Autodesk Fusion 360 part; units mm, degrees
note: some values were not read from the file. Set by a fixed rule: which sketch regions a step uses.
(part 2 of 3)
sketch "Sketch3" plane through (0, 0, 5) normal (0, 0, 1) x (-1, 0, 0)
  line L0 (-183.6113, -17.3326) -> (-182.6113, -19.0647)
  line L1 (-182.6113, -19.0647) -> (-183.6113, -20.7967)
  line L2 (-183.6113, -20.7967) -> (-179.9574, -28.2505)
  arc A0 (-179.9574, -28.2505) -> (-178.1615, -29.3702) centre (-178.1615, -27.3702) ccw
  line L3 (-178.1615, -29.3702) -> (-149.6323, -29.3702)
  line L4 (-149.6323, -29.3702) -> (-149.6323, -24.3702)
  line L5 (-149.6323, -24.3702) -> (-169.6572, -23.9078)
  arc A1 (-170.1456, -23.408) -> (-169.6572, -23.9078) centre (-169.6456, -23.408) ccw
  line L6 (-170.1456, -23.408) -> (-170.1456, -20.1187)
  arc A2 (-169.9247, -19.9198) -> (-170.1456, -20.1187) centre (-169.9456, -20.1187) ccw
  line L7 (-169.9247, -19.9198) -> (-167.3247, -20.1931)
  arc A3 (-167.1456, -20.392) -> (-167.3247, -20.1931) centre (-167.3456, -20.392) ccw
  line L8 (-167.1456, -20.392) -> (-167.1456, -20.5119)
  line L9 (-167.1456, -20.5119) -> (-151.6323, -22.1424)
  line L10 (-151.6323, -22.1424) -> (-151.6323, -22.0645)
  arc A4 (-151.4114, -21.8656) -> (-151.6323, -22.0645) centre (-151.4323, -22.0645) ccw
  line L11 (-151.4114, -21.8656) -> (-148.8114, -22.1389)
  arc A5 (-148.6323, -22.3378) -> (-148.8114, -22.1389) centre (-148.8323, -22.3378) ccw
  line L12 (-148.6323, -22.3378) -> (-148.6323, -33.3702)
  arc A6 (-149.1323, -33.8702) -> (-148.6323, -33.3702) centre (-149.1323, -33.3702) ccw
  line L13 (-149.1323, -33.8702) -> (-150.6323, -33.8702)
  arc A7 (-150.6323, -33.8702) -> (-151.1323, -34.3702) centre (-150.6323, -34.3702) ccw
  line L14 (-151.1323, -34.3702) -> (-151.1323, -38.0378)
  arc A8 (-151.1323, -38.0378) -> (-150.4871, -38.5162) centre (-150.6323, -38.0378) ccw
  arc A9 (-141.7774, -38.5162) -> (-150.4871, -38.5162) centre (-146.1323, -52.8702) ccw
  arc A10 (-141.7774, -38.5162) -> (-141.1323, -38.0378) centre (-141.6323, -38.0378) ccw
  line L15 (-141.1323, -38.0378) -> (-141.1323, -34.3702)
  arc A11 (-141.1323, -34.3702) -> (-141.6323, -33.8702) centre (-141.6323, -34.3702) ccw
  line L16 (-141.6323, -33.8702) -> (-143.1323, -33.8702)
  arc A12 (-143.6323, -33.3702) -> (-143.1323, -33.8702) centre (-143.1323, -33.3702) ccw
  line L17 (-143.6323, -33.3702) -> (-143.6323, -22.3378)
  arc A13 (-143.4532, -22.1389) -> (-143.6323, -22.3378) centre (-143.4323, -22.3378) ccw
  line L18 (-143.4532, -22.1389) -> (-140.6323, -21.8424)
  line L19 (-140.6323, -21.8424) -> (-140.6323, -21.9203)
  arc A14 (-140.6323, -21.9203) -> (-140.4114, -22.1192) centre (-140.4323, -21.9203) ccw
  line L20 (-140.4114, -22.1192) -> (-125.298, -20.5307)
  arc A15 (-125.298, -20.5307) -> (-125.1189, -20.3318) centre (-125.3189, -20.3318) ccw
  line L21 (-125.1189, -20.3318) -> (-125.1189, -20.3019)
  arc A16 (-125.0294, -20.2025) -> (-125.1189, -20.3019) centre (-125.0189, -20.3019) ccw
  line L22 (-125.0294, -20.2025) -> (-122.3398, -19.9198)
  arc A17 (-122.1189, -20.1187) -> (-122.3398, -19.9198) centre (-122.3189, -20.1187) ccw
  line L23 (-122.1189, -20.1187) -> (-122.1189, -23.408)
  arc A18 (-122.6074, -23.9078) -> (-122.1189, -23.408) centre (-122.6189, -23.408) ccw
  line L24 (-122.6074, -23.9078) -> (-142.1438, -24.3589)
  line L25 (-142.1438, -24.3589) -> (-142.6323, -24.3589)
  line L26 (-142.6323, -24.3589) -> (-142.6323, -29.3702)
  line L27 (-142.6323, -29.3702) -> (-117.7597, -29.3702)
  arc A19 (-117.7597, -29.3702) -> (-113.1229, -26.2409) centre (-117.7597, -24.3702) ccw
  arc A20 (-89.3732, -10.2649) -> (-113.1229, -26.2409) centre (-89.45, -35.7917) ccw
  line L28 (-89.3732, -10.2649) -> (-11.704, -12.452)
  arc A21 (-11.704, -12.452) -> (-11.9433, 12.5645) centre (-11.002, 0.0641) ccw
  line L29 (-11.9433, 12.5645) -> (-80.6073, 9.9709)
  arc A22 (-112.7407, 25.7315) -> (-80.6073, 9.9709) centre (-80.1774, 51.4853) ccw
  arc A23 (-112.7407, 25.7315) -> (-116.6624, 27.6298) centre (-116.6624, 22.6298) ccw
  line L30 (-116.6624, 27.6298) -> (-197.169, 27.6298)
  arc A24 (-197.169, 27.6298) -> (-202.169, 22.6429) centre (-197.169, 22.6298) ccw
  line L31 (-202.169, 22.6429) -> (-202.2039, 9.25)
  line L32 (-202.2039, 9.25) -> (-186.5961, 9.1821)
  arc A25 (-186.5961, 9.1821) -> (-186.1089, 9.5607) centre (-186.5939, 9.6821) ccw
  line L33 (-186.1089, 9.5607) -> (-182.6828, 23.2512)
  arc A26 (-182.1978, 23.6298) -> (-182.6828, 23.2512) centre (-182.1978, 23.1298) ccw
  line L34 (-182.1978, 23.6298) -> (-178.088, 23.6298)
  arc A27 (-177.588, 23.1298) -> (-178.088, 23.6298) centre (-178.088, 23.1298) ccw
  line L35 (-177.588, 23.1298) -> (-177.588, 7.1298)
  arc A28 (-178.088, 6.6298) -> (-177.588, 7.1298) centre (-178.088, 7.1298) ccw
  line L36 (-178.088, 6.6298) -> (-185.5859, 6.6298)
  arc A29 (-186.0859, 7.132) -> (-185.5859, 6.6298) centre (-185.5859, 7.1298) ccw
  line L37 (-186.0859, 7.132) -> (-186.0802, 8.4298)
  arc A30 (-186.0802, 8.4298) -> (-186.578, 8.932) centre (-186.5802, 8.432) ccw
  line L38 (-186.578, 8.932) -> (-202.156, 8.9998)
  line L39 (-202.156, 8.9998) -> (-202.156, -24.3702)
  arc A31 (-202.156, -24.3702) -> (-197.156, -29.3702) centre (-197.156, -24.3702) ccw
  line L40 (-197.156, -29.3702) -> (-190.889, -29.3702)
  arc A32 (-190.889, -29.3702) -> (-189.0932, -28.2505) centre (-190.889, -27.3702) ccw
  line L41 (-189.0932, -28.2505) -> (-185.4393, -20.7967)
  line L42 (-185.4393, -20.7967) -> (-186.4393, -19.0647)
  line L43 (-186.4393, -19.0647) -> (-185.4393, -17.3326)
  line L44 (-185.4393, -17.3326) -> (-186.4393, -15.6006)
  line L45 (-186.4393, -15.6006) -> (-185.4393, -13.8685)
  line L46 (-185.4393, -13.8685) -> (-186.4393, -12.1365)
  line L47 (-186.4393, -12.1365) -> (-185.4393, -10.4044)
  line L48 (-185.4393, -10.4044) -> (-186.4393, -8.6724)
  line L49 (-186.4393, -8.6724) -> (-185.4393, -6.9403)
  line L50 (-185.4393, -6.9403) -> (-186.4393, -5.2083)
  line L51 (-186.4393, -5.2083) -> (-185.4393, -3.4762)
  line L52 (-185.4393, -3.4762) -> (-186.4393, -1.7442)
  line L53 (-186.4393, -1.7442) -> (-185.4592, -0.0467)
  line L54 (-185.4592, -0.0467) -> (-185.4592, 2.1298)
  arc A33 (-184.9592, 2.6298) -> (-185.4592, 2.1298) centre (-184.9592, 2.1298) ccw
  line L55 (-184.9592, 2.6298) -> (-165.8788, 2.6298)
  arc A34 (-165.8788, 2.6298) -> (-165.3864, 3.043) centre (-165.8788, 3.1298) ccw
  line L56 (-165.3864, 3.043) -> (-162.9139, 17.0652)
  arc A35 (-162.4215, 17.4784) -> (-162.9139, 17.0652) centre (-162.4215, 16.9784) ccw
  line L57 (-162.4215, 17.4784) -> (-161.7176, 17.4784)
  arc A36 (-161.2489, 17.1526) -> (-161.7176, 17.4784) centre (-161.7176, 16.9784) ccw
  spline S0 degree 5 poles (-161.2489, 17.1526) (-161.0282, 16.559) (-160.5594, 15.3025) (-159.8388, 13.3845) (-158.8598, 10.8079) (-157.6127, 7.5765) (-156.3196, 4.2834) (-155.0058, 0.9987) (-153.6703, -2.2771) (-152.3141, -5.5444) (-150.9388, -8.8038) (-149.8244, -11.4057) (-148.9812, -13.354) (-148.4158, -14.6516) (-148.1323, -15.3) knots -0.989467 -0.989467 -0.989467 -0.989467 -0.989467 -0.989467 -0.9 -0.8 -0.7 -0.6 -0.5 -0.4 -0.3 -0.2 -0.1 0 0 0 0 0 0
  line L58 (-148.1323, -15.3) -> (-148.3823, -15.3)
  arc A37 (-148.3823, -15.3) -> (-148.6323, -15.55) centre (-148.3823, -15.55) ccw
  line L59 (-148.6323, -15.55) -> (-148.6323, -17.4356)
  arc A38 (-148.8532, -17.6345) -> (-148.6323, -17.4356) centre (-148.8323, -17.4356) ccw
  line L60 (-148.8532, -17.6345) -> (-151.4532, -17.3612)
  arc A39 (-151.6323, -17.1623) -> (-151.4532, -17.3612) centre (-151.4323, -17.1623) ccw
  line L61 (-151.6323, -17.1623) -> (-151.6323, -17.0424)
  line L62 (-151.6323, -17.0424) -> (-167.1456, -15.4119)
  line L63 (-167.1456, -15.4119) -> (-167.1456, -15.4898)
  arc A40 (-167.3665, -15.6887) -> (-167.1456, -15.4898) centre (-167.3456, -15.4898) ccw
  line L64 (-167.3665, -15.6887) -> (-169.9665, -15.4154)
  arc A41 (-170.1456, -15.2165) -> (-169.9665, -15.4154) centre (-169.9456, -15.2165) ccw
  line L65 (-170.1456, -15.2165) -> (-170.1456, -13.9739)
  arc A42 (-170.1456, -13.9739) -> (-170.6456, -13.1079) centre (-171.1456, -13.9739) ccw
  line L66 (-170.6456, -13.1079) -> (-173.5, -11.4599)
  arc A43 (-176, -7.1298) -> (-173.5, -11.4599) centre (-171, -7.1298) ccw
  line L67 (-176, -7.1298) -> (-176, 1.6298)
  line L68 (-176, 1.6298) -> (-183.6113, 1.6298)
  line L69 (-183.6113, 1.6298) -> (-183.6113, -0.0121)
  line L70 (-183.6113, -0.0121) -> (-182.6113, -1.7442)
  line L71 (-182.6113, -1.7442) -> (-183.6113, -3.4762)
  line L72 (-183.6113, -3.4762) -> (-182.6113, -5.2083)
  line L73 (-182.6113, -5.2083) -> (-183.6113, -6.9403)
  line L74 (-183.6113, -6.9403) -> (-182.6113, -8.6724)
  line L75 (-182.6113, -8.6724) -> (-183.6113, -10.4044)
  line L76 (-183.6113, -10.4044) -> (-182.6113, -12.1365)
  line L77 (-182.6113, -12.1365) -> (-183.6113, -13.8685)
  line L78 (-183.6113, -13.8685) -> (-182.6113, -15.6006)
  line L79 (-182.6113, -15.6006) -> (-183.6113, -17.3326)
  arc A44 (-143.6323, -21.4356) -> (-143.4114, -21.6345) centre (-143.4323, -21.4356) ccw
  line L80 (-143.6323, -21.4356) -> (-143.6323, -20.3378)
  arc A45 (-143.4532, -20.1389) -> (-143.6323, -20.3378) centre (-143.4323, -20.3378) ccw
  line L81 (-143.4532, -20.1389) -> (-140.6323, -19.8424)
  line L82 (-140.6323, -19.8424) -> (-140.6323, -19.9203)
  arc A46 (-140.6323, -19.9203) -> (-140.4114, -20.1192) centre (-140.4323, -19.9203) ccw
  line L83 (-140.4114, -20.1192) -> (-125.298, -18.5307)
  arc A47 (-125.298, -18.5307) -> (-125.1189, -18.3318) centre (-125.3189, -18.3318) ccw
  line L84 (-125.1189, -18.3318) -> (-125.1189, -18.2119)
  line L85 (-125.1189, -18.2119) -> (-122.3398, -17.9198)
  arc A48 (-122.1189, -18.1187) -> (-122.3398, -17.9198) centre (-122.3189, -18.1187) ccw
  line L86 (-122.1189, -18.1187) -> (-122.1189, -19.2165)
  arc A49 (-122.298, -19.4154) -> (-122.1189, -19.2165) centre (-122.3189, -19.2165) ccw
  line L87 (-122.298, -19.4154) -> (-125.1189, -19.7119)
  line L88 (-125.1189, -19.7119) -> (-125.1189, -19.634)
  arc A50 (-125.1189, -19.634) -> (-125.3398, -19.4351) centre (-125.3189, -19.634) ccw
  line L89 (-125.3398, -19.4351) -> (-140.4532, -21.0236)
  arc A51 (-140.4532, -21.0236) -> (-140.6323, -21.2225) centre (-140.4323, -21.2225) ccw
  line L90 (-140.6323, -21.2225) -> (-140.6323, -21.2524)
  arc A52 (-140.7218, -21.3518) -> (-140.6323, -21.2524) centre (-140.7323, -21.2524) ccw
  line L91 (-140.7218, -21.3518) -> (-143.4114, -21.6345)
  arc A53 (-143.6323, -19.4356) -> (-143.4114, -19.6345) centre (-143.4323, -19.4356) ccw
  line L92 (-143.6323, -19.4356) -> (-143.6323, -18.3378)
  arc A54 (-143.4532, -18.1389) -> (-143.6323, -18.3378) centre (-143.4323, -18.3378) ccw
  line L93 (-143.4532, -18.1389) -> (-140.6323, -17.8424)
  line L94 (-140.6323, -17.8424) -> (-140.6323, -17.9203)
  arc A55 (-140.6323, -17.9203) -> (-140.4114, -18.1192) centre (-140.4323, -17.9203) ccw
  line L95 (-140.4114, -18.1192) -> (-125.298, -16.5307)
  arc A56 (-125.298, -16.5307) -> (-125.1189, -16.3318) centre (-125.3189, -16.3318) ccw
  line L96 (-125.1189, -16.3318) -> (-125.1189, -16.2119)
  line L97 (-125.1189, -16.2119) -> (-122.3398, -15.9198)
  arc A57 (-122.1189, -16.1187) -> (-122.3398, -15.9198) centre (-122.3189, -16.1187) ccw
  line L98 (-122.1189, -16.1187) -> (-122.1189, -17.2165)
  arc A58 (-122.298, -17.4154) -> (-122.1189, -17.2165) centre (-122.3189, -17.2165) ccw
  line L99 (-122.298, -17.4154) -> (-125.1189, -17.7119)
  line L100 (-125.1189, -17.7119) -> (-125.1189, -17.634)
  arc A59 (-125.1189, -17.634) -> (-125.3398, -17.4351) centre (-125.3189, -17.634) ccw
  line L101 (-125.3398, -17.4351) -> (-140.4532, -19.0236)
  arc A60 (-140.4532, -19.0236) -> (-140.6323, -19.2225) centre (-140.4323, -19.2225) ccw
  line L102 (-140.6323, -19.2225) -> (-140.6323, -19.2524)
  arc A61 (-140.7218, -19.3518) -> (-140.6323, -19.2524) centre (-140.7323, -19.2524) ccw
  line L103 (-140.7218, -19.3518) -> (-143.4114, -19.6345)
  arc A62 (-123.4224, 7.043) -> (-122.93, 6.6298) centre (-122.93, 7.1298) ccw
  line L104 (-123.4224, 7.043) -> (-126.0097, 21.7167)
  arc A63 (-126.0097, 21.7167) -> (-126.5021, 22.1298) centre (-126.5021, 21.6298) ccw
  line L105 (-126.5021, 22.1298) -> (-165.663, 22.1298)
  arc A64 (-165.663, 22.1298) -> (-166.1554, 21.7167) centre (-165.663, 21.6298) ccw
  line L106 (-166.1554, 21.7167) -> (-168.7428, 7.043)
  arc A65 (-169.2352, 6.6298) -> (-168.7428, 7.043) centre (-169.2352, 7.1298) ccw
  line L107 (-169.2352, 6.6298) -> (-176.588, 6.6298)
  arc A66 (-177.088, 7.1298) -> (-176.588, 6.6298) centre (-176.588, 7.1298) ccw
  line L108 (-177.088, 7.1298) -> (-177.088, 23.1298)
  arc A67 (-176.588, 23.6298) -> (-177.088, 23.1298) centre (-176.588, 23.1298) ccw
  line L109 (-176.588, 23.6298) -> (-121.7059, 23.6298)
  arc A68 (-121.2059, 23.1298) -> (-121.7059, 23.6298) centre (-121.7059, 23.1298) ccw
  line L110 (-121.2059, 23.1298) -> (-121.2059, 7.1298)
  arc A69 (-121.7059, 6.6298) -> (-121.2059, 7.1298) centre (-121.7059, 7.1298) ccw
  line L111 (-121.7059, 6.6298) -> (-122.93, 6.6298)
  line L112 (-167.1456, -16.5119) -> (-151.6323, -18.1424)
  line L113 (-151.6323, -18.1424) -> (-151.6323, -18.0645)
  arc A70 (-151.4114, -17.8656) -> (-151.6323, -18.0645) centre (-151.4323, -18.0645) ccw
  line L114 (-151.4114, -17.8656) -> (-148.8114, -18.1389)
  arc A71 (-148.6323, -18.3378) -> (-148.8114, -18.1389) centre (-148.8323, -18.3378) ccw
  line L115 (-148.6323, -18.3378) -> (-148.6323, -19.4356)
  arc A72 (-148.8532, -19.6345) -> (-148.6323, -19.4356) centre (-148.8323, -19.4356) ccw
  line L116 (-148.8532, -19.6345) -> (-151.4532, -19.3612)
  arc A73 (-151.6323, -19.1623) -> (-151.4532, -19.3612) centre (-151.4323, -19.1623) ccw
  line L117 (-151.6323, -19.1623) -> (-151.6323, -19.0424)
  line L118 (-151.6323, -19.0424) -> (-167.1456, -17.4119)
  line L119 (-167.1456, -17.4119) -> (-167.1456, -17.4898)
  arc A74 (-167.3665, -17.6887) -> (-167.1456, -17.4898) centre (-167.3456, -17.4898) ccw
  line L120 (-167.3665, -17.6887) -> (-169.9665, -17.4154)
  arc A75 (-170.1456, -17.2165) -> (-169.9665, -17.4154) centre (-169.9456, -17.2165) ccw
  line L121 (-170.1456, -17.2165) -> (-170.1456, -16.1187)
  arc A76 (-169.9247, -15.9198) -> (-170.1456, -16.1187) centre (-169.9456, -16.1187) ccw
  line L122 (-169.9247, -15.9198) -> (-167.3247, -16.1931)
  arc A77 (-167.1456, -16.392) -> (-167.3247, -16.1931) centre (-167.3456, -16.392) ccw
  line L123 (-167.1456, -16.392) -> (-167.1456, -16.5119)
  spline S1 degree 5 poles (-131.6523, 17.4499) (-131.871, 16.8829) (-132.3693, 15.5934) (-133.1481, 13.5859) (-134.2095, 10.8681) (-135.5564, 7.4521) (-136.9701, 3.9054) (-138.3903, 0.385) (-139.8173, -3.108) (-141.2507, -6.5745) (-142.5604, -9.7063) (-143.5856, -12.1354) (-144.3238, -13.8732) (-144.7729, -14.9268) (-144.9323, -15.3) knots -0.978339 -0.978339 -0.978339 -0.978339 -0.978339 -0.978339 -0.9 -0.8 -0.7 -0.6 -0.5 -0.4 -0.3 -0.2 -0.1 -0.045074 -0.045074 -0.045074 -0.045074 -0.045074 -0.045074
  line L124 (-144.9323, -15.3) -> (-147.3323, -15.3)
  spline S2 degree 3 poles (-147.3323, -15.3) (-147.3606, -15.2315) (-147.3889, -15.163) (-147.4174, -15.0945) (-147.7999, -14.1733) (-148.2003, -13.2596) (-148.603, -12.3469) (-149.0343, -11.3694) (-149.4682, -10.3932) (-149.9035, -9.4176) (-150.1094, -8.9559) (-150.3157, -8.4943) (-150.5222, -8.0328) knots 80.396364 80.396364 80.396364 80.396364 80.841267 80.841267 80.841267 86.826165 86.826165 86.826165 93.23622 93.23622 93.23622 96.269727 96.269727 96.269727 96.269727
  spline S3 degree 5 poles (-150.5222, -8.0328) (-150.5836, -7.8891) (-150.9212, -7.0983) (-151.5369, -5.6459) (-152.4351, -3.5002) (-153.6231, -0.6091) (-155.0461, 2.9325) (-156.4844, 6.5848) (-157.7568, 9.8732) (-158.7459, 12.4635) (-159.4459, 14.3123) (-159.8529, 15.3927) (-159.9652, 15.6911) knots -0.722257 -0.722257 -0.722257 -0.722257 -0.722257 -0.722257 -0.7 -0.6 -0.5 -0.4 -0.3 -0.2 -0.1 -0.061951 -0.061951 -0.061951 -0.061951 -0.061951 -0.061951
  line L125 (-159.9652, 15.6911) -> (-160.6285, 17.4538)
  arc A78 (-160.1605, 18.1298) -> (-160.6285, 17.4538) centre (-160.1605, 17.6298) ccw
  line L126 (-160.1605, 18.1298) -> (-132.1188, 18.1298)
  arc A79 (-131.6523, 17.4499) -> (-132.1188, 18.1298) centre (-132.1188, 17.6298) ccw
  arc A80 (-143.6323, -17.4356) -> (-143.4114, -17.6345) centre (-143.4323, -17.4356) ccw
  line L127 (-143.6323, -17.4356) -> (-143.6323, -15.55)
  arc A81 (-143.6323, -15.55) -> (-143.8823, -15.3) centre (-143.8823, -15.55) ccw
  line L128 (-143.8823, -15.3) -> (-144.1323, -15.3)
  spline S4 degree 5 poles (-144.1323, -15.3) (-144.0034, -15.0117) (-143.5692, -14.0387) (-142.8329, -12.3782) (-141.8006, -10.0246) (-140.482, -6.9691) (-139.0131, -3.4934) (-137.5684, 0.0041) (-136.1486, 3.5243) (-134.7528, 7.0662) (-133.3923, 10.5941) (-132.3224, 13.424) (-131.5314, 15.5453) (-131.012, 16.9513) (-130.7595, 17.6378) knots -0.94214 -0.94214 -0.94214 -0.94214 -0.94214 -0.94214 -0.9 -0.8 -0.7 -0.6 -0.5 -0.4 -0.3 -0.2 -0.1 -0.004792 -0.004792 -0.004792 -0.004792 -0.004792 -0.004792
  line L129 (-130.7595, 17.6378) -> (-129.7718, 17.6378)
  arc A82 (-129.2794, 17.2246) -> (-129.7718, 17.6378) centre (-129.7718, 17.1378) ccw
  line L130 (-129.2794, 17.2246) -> (-126.7788, 3.043)
  arc A83 (-126.7788, 3.043) -> (-126.2864, 2.6298) centre (-126.2864, 3.1298) ccw
  line L131 (-126.2864, 2.6298) -> (-120.2059, 2.6298)
  arc A84 (-120.2059, 2.6298) -> (-119.7059, 3.1298) centre (-120.2059, 3.1298) ccw
  line L132 (-119.7059, 3.1298) -> (-119.7059, 6.1298)
  arc A85 (-119.7059, 6.1298) -> (-120.2059, 6.6298) centre (-120.2059, 6.1298) ccw
  arc A86 (-120.7059, 7.1298) -> (-120.2059, 6.6298) centre (-120.2059, 7.1298) ccw
  line L133 (-120.7059, 7.1298) -> (-120.7059, 23.1298)
  arc A87 (-120.2059, 23.6298) -> (-120.7059, 23.1298) centre (-120.2059, 23.1298) ccw
  line L134 (-120.2059, 23.6298) -> (-118.121, 23.6298)
  arc A88 (-117.6301, 23.2247) -> (-118.121, 23.6298) centre (-118.121, 23.1298) ccw
  line L135 (-117.6301, 23.2247) -> (-115.2816, 11.0735)
  line L136 (-115.1907, 10.1247) -> (-115.1907, -6.5098)
  arc A89 (-117.6907, -10.8399) -> (-115.1907, -6.5098) centre (-120.1907, -6.5098) ccw
  line L137 (-117.6907, -10.8399) -> (-121.6189, -13.1079)
  arc A90 (-121.6189, -13.1079) -> (-122.1189, -13.9739) centre (-121.1189, -13.9739) ccw
  line L138 (-122.1189, -13.9739) -> (-122.1189, -15.2165)
  arc A91 (-122.298, -15.4154) -> (-122.1189, -15.2165) centre (-122.3189, -15.2165) ccw
  line L139 (-122.298, -15.4154) -> (-125.1189, -15.7119)
  line L140 (-125.1189, -15.7119) -> (-125.1189, -15.634)
  arc A92 (-125.1189, -15.634) -> (-125.3398, -15.4351) centre (-125.3189, -15.634) ccw
  line L141 (-125.3398, -15.4351) -> (-140.4532, -17.0236)
  arc A93 (-140.4532, -17.0236) -> (-140.6323, -17.2225) centre (-140.4323, -17.2225) ccw
  line L142 (-140.6323, -17.2225) -> (-140.6323, -17.1623)
  arc A94 (-140.8114, -17.3612) -> (-140.6323, -17.1623) centre (-140.8323, -17.1623) ccw
  line L143 (-140.8114, -17.3612) -> (-143.4114, -17.6345)
  line L144 (-167.1456, -18.5119) -> (-151.6323, -20.1424)
  line L145 (-151.6323, -20.1424) -> (-151.6323, -20.0645)
  arc A95 (-151.4114, -19.8656) -> (-151.6323, -20.0645) centre (-151.4323, -20.0645) ccw
  line L146 (-151.4114, -19.8656) -> (-148.8114, -20.1389)
  arc A96 (-148.6323, -20.3378) -> (-148.8114, -20.1389) centre (-148.8323, -20.3378) ccw
  line L147 (-148.6323, -20.3378) -> (-148.6323, -21.4356)
  arc A97 (-148.8532, -21.6345) -> (-148.6323, -21.4356) centre (-148.8323, -21.4356) ccw
  line L148 (-148.8532, -21.6345) -> (-151.4532, -21.3612)
  arc A98 (-151.6323, -21.1623) -> (-151.4532, -21.3612) centre (-151.4323, -21.1623) ccw
  line L149 (-151.6323, -21.1623) -> (-151.6323, -21.0424)
  line L150 (-151.6323, -21.0424) -> (-167.1456, -19.4119)
  line L151 (-167.1456, -19.4119) -> (-167.1456, -19.4898)
  arc A99 (-167.3665, -19.6887) -> (-167.1456, -19.4898) centre (-167.3456, -19.4898) ccw
  line L152 (-167.3665, -19.6887) -> (-169.9665, -19.4154)
  arc A100 (-170.1456, -19.2165) -> (-169.9665, -19.4154) centre (-169.9456, -19.2165) ccw
  line L153 (-170.1456, -19.2165) -> (-170.1456, -18.1187)
  arc A101 (-169.9247, -17.9198) -> (-170.1456, -18.1187) centre (-169.9456, -18.1187) ccw
  line L154 (-169.9247, -17.9198) -> (-167.3247, -18.1931)
  arc A102 (-167.1456, -18.392) -> (-167.3247, -18.1931) centre (-167.3456, -18.392) ccw
  line L155 (-167.1456, -18.392) -> (-167.1456, -18.5119)
  circle A103 centre (-11.002, 0.0641) radius 7.5
  line L156 (-126.9683, -24.0085) -> (-126.9683, -29.3702)
  line L157 (-164.0862, -24.0085) -> (-164.0862, -29.3702)
  line L158 (-182.6113, -5.2083) -> (-178.6113, -5.2083)
  line L159 (-178.6113, -5.2083) -> (-178.6113, 1.6298)
  arc A104 (-115.1907, 10.1247) -> (-115.2816, 11.0735) centre (-120.1907, 10.1247) ccw
  dimension "d155" = 5
  constraint coincident L24 L156.start
  constraint coincident L27 L156.end
  constraint perpendicular L27 L156
  constraint coincident L3 L157.end
  constraint perpendicular L3 L157
  constraint coincident L72.end L73.start
  constraint perpendicular L67 L158
  constraint coincident L68 L159.end
  constraint perpendicular L68 L159
  measures "d155" distance of L69 L159
extrude "Extrude2" add sketch "Sketch3" along normal blind 2 contours L3 L4 L5 L157 | L68 L69 L70 L71 L72 L158 L159 | L24 L25 L26 L27 L156
sketch "Sketch4" plane through (0, -1.6298, 0) normal (0, -1, 0) x (1, 0, 0)
  line L0 (176, 0) -> (183.6113, 0)
  line L1 (183.6113, 0) -> (183.6113, 7)
  line L2 (183.6113, 7) -> (178.6113, 7)
  line L3 (178.6113, 7) -> (178.6113, 5)
  line L4 (178.6113, 5) -> (176, 5)
  line L5 (176, 5) -> (176, 0)
  line L6 (178.6113, 7) -> (183.6113, 7)
  line L7 (183.6113, 7) -> (183.6113, 5.3)
  line L8 (183.6113, 5.3) -> (178.6113, 5.3)
  line L9 (178.6113, 5.3) -> (178.6113, 7)
  dimension "d156" = 1.7
  constraint horizontal L6
  constraint vertical L7
  constraint horizontal L8
  constraint vertical L9
  constraint coincident L2.end L3.start
  measures "d156" distance of L2.end L8.end
sketch "Sketch5" plane through (149.6323, 0, 0) normal (-1, 0, 0) x (0, -1, 0)
  line L0 (-29.3702, 0) -> (-24.3702, 0)
  line L1 (-24.3702, 0) -> (-24.3702, 7)
  line L2 (-24.3702, 7) -> (-29.3702, 7)
  line L3 (-29.3702, 7) -> (-29.3702, 0)
  line L4 (-29.3702, 7) -> (-24.3702, 7)
  line L5 (-24.3702, 7) -> (-24.3702, 5.3)
  line L6 (-24.3702, 5.3) -> (-29.3702, 5.3)
  line L7 (-29.3702, 5.3) -> (-29.3702, 7)
  dimension "d157" = 1.7
  constraint horizontal L4
  constraint vertical L5
  constraint horizontal L6
  constraint vertical L7
  constraint coincident L2.end L3.start
  measures "d157" distance of L2.end L6.end
extrude "Extrude3" add sketch "Sketch5" along normal blind 7 contours L1 L2 L3 L4 L5 L6 L7
extrude "Extrude4" add sketch "Sketch4" along normal blind 26 contours L1 L2 L3 L6 L7 L8 L9
sketch "Sketch6" plane through (0, 0, 5) normal (0, 0, 1) x (-1, 0, 0)
  line L0 (-178.6113, 1.6298) -> (-178.6113, -5.2083)
  line L1 (-178.6113, -5.2083) -> (-182.6113, -5.2083)
  line L2 (-182.6113, -5.2083) -> (-183.6113, -6.9403)
  line L3 (-183.6113, -6.9403) -> (-182.6113, -8.6724)
  line L4 (-182.6113, -8.6724) -> (-183.6113, -10.4044)
  line L5 (-183.6113, -10.4044) -> (-182.6113, -12.1365)
  line L6 (-182.6113, -12.1365) -> (-183.6113, -13.8685)
  line L7 (-183.6113, -13.8685) -> (-182.6113, -15.6006)
  line L8 (-182.6113, -15.6006) -> (-183.6113, -17.3326)
  line L9 (-183.6113, -17.3326) -> (-182.6113, -19.0647)
  line L10 (-182.6113, -19.0647) -> (-183.6113, -20.7967)
  line L11 (-183.6113, -20.7967) -> (-179.9574, -28.2505)
  arc A0 (-179.9574, -28.2505) -> (-178.1615, -29.3702) centre (-178.1615, -27.3702) ccw
  line L12 (-178.1615, -29.3702) -> (-164.0862, -29.3702)
  line L13 (-164.0862, -29.3702) -> (-164.0862, -24.0365)
  line L14 (-164.0862, -24.0365) -> (-169.6572, -23.9078)
  arc A1 (-170.1456, -23.408) -> (-169.6572, -23.9078) centre (-169.6456, -23.408) ccw
  line L15 (-170.1456, -23.408) -> (-170.1456, -20.1187)
  arc A2 (-169.9247, -19.9198) -> (-170.1456, -20.1187) centre (-169.9456, -20.1187) ccw
  line L16 (-169.9247, -19.9198) -> (-167.3247, -20.1931)
  arc A3 (-167.1456, -20.392) -> (-167.3247, -20.1931) centre (-167.3456, -20.392) ccw
  line L17 (-167.1456, -20.392) -> (-167.1456, -20.5119)
  line L18 (-167.1456, -20.5119) -> (-151.6323, -22.1424)
  line L19 (-151.6323, -22.1424) -> (-151.6323, -22.0645)
  arc A4 (-151.4114, -21.8656) -> (-151.6323, -22.0645) centre (-151.4323, -22.0645) ccw
  line L20 (-151.4114, -21.8656) -> (-148.8114, -22.1389)
  arc A5 (-148.6323, -22.3378) -> (-148.8114, -22.1389) centre (-148.8323, -22.3378) ccw
  line L21 (-148.6323, -22.3378) -> (-148.6323, -33.3702)
  arc A6 (-149.1323, -33.8702) -> (-148.6323, -33.3702) centre (-149.1323, -33.3702) ccw
  line L22 (-149.1323, -33.8702) -> (-150.6323, -33.8702)
  arc A7 (-150.6323, -33.8702) -> (-151.1323, -34.3702) centre (-150.6323, -34.3702) ccw
  line L23 (-151.1323, -34.3702) -> (-151.1323, -38.0378)
  arc A8 (-151.1323, -38.0378) -> (-150.4871, -38.5162) centre (-150.6323, -38.0378) ccw
  arc A9 (-141.7774, -38.5162) -> (-150.4871, -38.5162) centre (-146.1323, -52.8702) ccw
  arc A10 (-141.7774, -38.5162) -> (-141.1323, -38.0378) centre (-141.6323, -38.0378) ccw
  line L24 (-141.1323, -38.0378) -> (-141.1323, -34.3702)
  arc A11 (-141.1323, -34.3702) -> (-141.6323, -33.8702) centre (-141.6323, -34.3702) ccw
  line L25 (-141.6323, -33.8702) -> (-143.1323, -33.8702)
  arc A12 (-143.6323, -33.3702) -> (-143.1323, -33.8702) centre (-143.1323, -33.3702) ccw
  line L26 (-143.6323, -33.3702) -> (-143.6323, -22.3378)
  arc A13 (-143.4532, -22.1389) -> (-143.6323, -22.3378) centre (-143.4323, -22.3378) ccw
  line L27 (-143.4532, -22.1389) -> (-140.6323, -21.8424)
  line L28 (-140.6323, -21.8424) -> (-140.6323, -21.9203)
  arc A14 (-140.6323, -21.9203) -> (-140.4114, -22.1192) centre (-140.4323, -21.9203) ccw
  line L29 (-140.4114, -22.1192) -> (-125.298, -20.5307)
  arc A15 (-125.298, -20.5307) -> (-125.1189, -20.3318) centre (-125.3189, -20.3318) ccw
  line L30 (-125.1189, -20.3318) -> (-125.1189, -20.3019)
  arc A16 (-125.0294, -20.2025) -> (-125.1189, -20.3019) centre (-125.0189, -20.3019) ccw
  line L31 (-125.0294, -20.2025) -> (-122.3398, -19.9198)
  arc A17 (-122.1189, -20.1187) -> (-122.3398, -19.9198) centre (-122.3189, -20.1187) ccw
  line L32 (-122.1189, -20.1187) -> (-122.1189, -23.408)
  arc A18 (-122.6074, -23.9078) -> (-122.1189, -23.408) centre (-122.6189, -23.408) ccw
  line L33 (-122.6074, -23.9078) -> (-126.9683, -24.0085)
  line L34 (-126.9683, -24.0085) -> (-126.9683, -29.3702)
  line L35 (-126.9683, -29.3702) -> (-117.7597, -29.3702)
  arc A19 (-117.7597, -29.3702) -> (-113.1229, -26.2409) centre (-117.7597, -24.3702) ccw
  arc A20 (-89.3732, -10.2649) -> (-113.1229, -26.2409) centre (-89.45, -35.7917) ccw
  line L36 (-89.3732, -10.2649) -> (-11.704, -12.452)
  arc A21 (-11.704, -12.452) -> (-11.9433, 12.5645) centre (-11.002, 0.0641) ccw
  line L37 (-11.9433, 12.5645) -> (-80.6073, 9.9709)
  arc A22 (-112.7407, 25.7315) -> (-80.6073, 9.9709) centre (-80.1774, 51.4853) ccw
  arc A23 (-112.7407, 25.7315) -> (-116.6624, 27.6298) centre (-116.6624, 22.6298) ccw
  line L38 (-116.6624, 27.6298) -> (-197.169, 27.6298)
  arc A24 (-197.169, 27.6298) -> (-202.169, 22.6429) centre (-197.169, 22.6298) ccw
  line L39 (-202.169, 22.6429) -> (-202.2039, 9.25)
  line L40 (-202.2039, 9.25) -> (-186.5961, 9.1821)
  arc A25 (-186.5961, 9.1821) -> (-186.1089, 9.5607) centre (-186.5939, 9.6821) ccw
  line L41 (-186.1089, 9.5607) -> (-182.6828, 23.2512)
  arc A26 (-182.1978, 23.6298) -> (-182.6828, 23.2512) centre (-182.1978, 23.1298) ccw
  line L42 (-182.1978, 23.6298) -> (-178.088, 23.6298)
  arc A27 (-177.588, 23.1298) -> (-178.088, 23.6298) centre (-178.088, 23.1298) ccw
  line L43 (-177.588, 23.1298) -> (-177.588, 7.1298)
  arc A28 (-178.088, 6.6298) -> (-177.588, 7.1298) centre (-178.088, 7.1298) ccw
  line L44 (-178.088, 6.6298) -> (-185.5859, 6.6298)
  arc A29 (-186.0859, 7.132) -> (-185.5859, 6.6298) centre (-185.5859, 7.1298) ccw
  line L45 (-186.0859, 7.132) -> (-186.0802, 8.4298)
  arc A30 (-186.0802, 8.4298) -> (-186.578, 8.932) centre (-186.5802, 8.432) ccw
  line L46 (-186.578, 8.932) -> (-202.156, 8.9998)
  line L47 (-202.156, 8.9998) -> (-202.156, -24.3702)
  arc A31 (-202.156, -24.3702) -> (-197.156, -29.3702) centre (-197.156, -24.3702) ccw
  line L48 (-197.156, -29.3702) -> (-190.889, -29.3702)
  arc A32 (-190.889, -29.3702) -> (-189.0932, -28.2505) centre (-190.889, -27.3702) ccw
  line L49 (-189.0932, -28.2505) -> (-185.4393, -20.7967)
  line L50 (-185.4393, -20.7967) -> (-186.4393, -19.0647)
  line L51 (-186.4393, -19.0647) -> (-185.4393, -17.3326)
  line L52 (-185.4393, -17.3326) -> (-186.4393, -15.6006)
  line L53 (-186.4393, -15.6006) -> (-185.4393, -13.8685)
  line L54 (-185.4393, -13.8685) -> (-186.4393, -12.1365)
  line L55 (-186.4393, -12.1365) -> (-185.4393, -10.4044)
  line L56 (-185.4393, -10.4044) -> (-186.4393, -8.6724)
  line L57 (-186.4393, -8.6724) -> (-185.4393, -6.9403)
  line L58 (-185.4393, -6.9403) -> (-186.4393, -5.2083)
  line L59 (-186.4393, -5.2083) -> (-185.4393, -3.4762)
  line L60 (-185.4393, -3.4762) -> (-186.4393, -1.7442)
  line L61 (-186.4393, -1.7442) -> (-185.4592, -0.0467)
  line L62 (-185.4592, -0.0467) -> (-185.4592, 2.1298)
  arc A33 (-184.9592, 2.6298) -> (-185.4592, 2.1298) centre (-184.9592, 2.1298) ccw
  line L63 (-184.9592, 2.6298) -> (-165.8788, 2.6298)
  arc A34 (-165.8788, 2.6298) -> (-165.3864, 3.043) centre (-165.8788, 3.1298) ccw
  line L64 (-165.3864, 3.043) -> (-162.9139, 17.0652)
  arc A35 (-162.4215, 17.4784) -> (-162.9139, 17.0652) centre (-162.4215, 16.9784) ccw
  line L65 (-162.4215, 17.4784) -> (-161.7176, 17.4784)
  arc A36 (-161.2489, 17.1526) -> (-161.7176, 17.4784) centre (-161.7176, 16.9784) ccw
  spline S0 degree 5 poles (-161.2489, 17.1526) (-161.0282, 16.559) (-160.5594, 15.3025) (-159.8388, 13.3845) (-158.8598, 10.8079) (-157.6127, 7.5765) (-156.3196, 4.2834) (-155.0058, 0.9987) (-153.6703, -2.2771) (-152.3141, -5.5444) (-150.9388, -8.8038) (-149.8244, -11.4057) (-148.9812, -13.354) (-148.4158, -14.6516) (-148.1323, -15.3) knots -0.989467 -0.989467 -0.989467 -0.989467 -0.989467 -0.989467 -0.9 -0.8 -0.7 -0.6 -0.5 -0.4 -0.3 -0.2 -0.1 0 0 0 0 0 0
  line L66 (-148.1323, -15.3) -> (-148.3823, -15.3)
  arc A37 (-148.3823, -15.3) -> (-148.6323, -15.55) centre (-148.3823, -15.55) ccw
  line L67 (-148.6323, -15.55) -> (-148.6323, -17.4356)
  arc A38 (-148.8532, -17.6345) -> (-148.6323, -17.4356) centre (-148.8323, -17.4356) ccw
  line L68 (-148.8532, -17.6345) -> (-151.4532, -17.3612)
  arc A39 (-151.6323, -17.1623) -> (-151.4532, -17.3612) centre (-151.4323, -17.1623) ccw
  line L69 (-151.6323, -17.1623) -> (-151.6323, -17.0424)
  line L70 (-151.6323, -17.0424) -> (-167.1456, -15.4119)
  line L71 (-167.1456, -15.4119) -> (-167.1456, -15.4898)
  arc A40 (-167.3665, -15.6887) -> (-167.1456, -15.4898) centre (-167.3456, -15.4898) ccw
  line L72 (-167.3665, -15.6887) -> (-169.9665, -15.4154)
  arc A41 (-170.1456, -15.2165) -> (-169.9665, -15.4154) centre (-169.9456, -15.2165) ccw
  line L73 (-170.1456, -15.2165) -> (-170.1456, -13.9739)
  arc A42 (-170.1456, -13.9739) -> (-170.6456, -13.1079) centre (-171.1456, -13.9739) ccw
  line L74 (-170.6456, -13.1079) -> (-173.5, -11.4599)
  arc A43 (-176, -7.1298) -> (-173.5, -11.4599) centre (-171, -7.1298) ccw
  line L75 (-176, -7.1298) -> (-176, 1.6298)
  line L76 (-176, 1.6298) -> (-178.6113, 1.6298)
  circle A44 centre (-11.002, 0.0641) radius 7.5
  line L77 (-167.1456, -18.5119) -> (-151.6323, -20.1424)
  line L78 (-151.6323, -20.1424) -> (-151.6323, -20.0645)
  arc A45 (-151.4114, -19.8656) -> (-151.6323, -20.0645) centre (-151.4323, -20.0645) ccw
  line L79 (-151.4114, -19.8656) -> (-148.8114, -20.1389)
  arc A46 (-148.6323, -20.3378) -> (-148.8114, -20.1389) centre (-148.8323, -20.3378) ccw
  line L80 (-148.6323, -20.3378) -> (-148.6323, -21.4356)
  arc A47 (-148.8532, -21.6345) -> (-148.6323, -21.4356) centre (-148.8323, -21.4356) ccw
  line L81 (-148.8532, -21.6345) -> (-151.4532, -21.3612)
  arc A48 (-151.6323, -21.1623) -> (-151.4532, -21.3612) centre (-151.4323, -21.1623) ccw
  line L82 (-151.6323, -21.1623) -> (-151.6323, -21.0424)
  line L83 (-151.6323, -21.0424) -> (-167.1456, -19.4119)
  line L84 (-167.1456, -19.4119) -> (-167.1456, -19.4898)
  arc A49 (-167.3665, -19.6887) -> (-167.1456, -19.4898) centre (-167.3456, -19.4898) ccw
  line L85 (-167.3665, -19.6887) -> (-169.9665, -19.4154)
  arc A50 (-170.1456, -19.2165) -> (-169.9665, -19.4154) centre (-169.9456, -19.2165) ccw
  line L86 (-170.1456, -19.2165) -> (-170.1456, -18.1187)
  arc A51 (-169.9247, -17.9198) -> (-170.1456, -18.1187) centre (-169.9456, -18.1187) ccw
  line L87 (-169.9247, -17.9198) -> (-167.3247, -18.1931)
  arc A52 (-167.1456, -18.392) -> (-167.3247, -18.1931) centre (-167.3456, -18.392) ccw
  line L88 (-167.1456, -18.392) -> (-167.1456, -18.5119)
  arc A53 (-143.6323, -17.4356) -> (-143.4114, -17.6345) centre (-143.4323, -17.4356) ccw
  line L89 (-143.6323, -17.4356) -> (-143.6323, -15.55)
  arc A54 (-143.6323, -15.55) -> (-143.8823, -15.3) centre (-143.8823, -15.55) ccw
  line L90 (-143.8823, -15.3) -> (-144.1323, -15.3)
  spline S1 degree 5 poles (-144.1323, -15.3) (-144.0034, -15.0117) (-143.5692, -14.0387) (-142.8329, -12.3782) (-141.8006, -10.0246) (-140.482, -6.9691) (-139.0131, -3.4934) (-137.5684, 0.0041) (-136.1486, 3.5243) (-134.7528, 7.0662) (-133.3923, 10.5941) (-132.3224, 13.424) (-131.5314, 15.5453) (-131.012, 16.9513) (-130.7595, 17.6378) knots -0.94214 -0.94214 -0.94214 -0.94214 -0.94214 -0.94214 -0.9 -0.8 -0.7 -0.6 -0.5 -0.4 -0.3 -0.2 -0.1 -0.004792 -0.004792 -0.004792 -0.004792 -0.004792 -0.004792
  line L91 (-130.7595, 17.6378) -> (-129.7718, 17.6378)
  arc A55 (-129.2794, 17.2246) -> (-129.7718, 17.6378) centre (-129.7718, 17.1378) ccw
  line L92 (-129.2794, 17.2246) -> (-126.7788, 3.043)
  arc A56 (-126.7788, 3.043) -> (-126.2864, 2.6298) centre (-126.2864, 3.1298) ccw
  line L93 (-126.2864, 2.6298) -> (-120.2059, 2.6298)
  arc A57 (-120.2059, 2.6298) -> (-119.7059, 3.1298) centre (-120.2059, 3.1298) ccw
  line L94 (-119.7059, 3.1298) -> (-119.7059, 6.1298)
  arc A58 (-119.7059, 6.1298) -> (-120.2059, 6.6298) centre (-120.2059, 6.1298) ccw
  arc A59 (-120.7059, 7.1298) -> (-120.2059, 6.6298) centre (-120.2059, 7.1298) ccw
  line L95 (-120.7059, 7.1298) -> (-120.7059, 23.1298)
  arc A60 (-120.2059, 23.6298) -> (-120.7059, 23.1298) centre (-120.2059, 23.1298) ccw
  line L96 (-120.2059, 23.6298) -> (-118.121, 23.6298)
  arc A61 (-117.6301, 23.2247) -> (-118.121, 23.6298) centre (-118.121, 23.1298) ccw
  line L97 (-117.6301, 23.2247) -> (-115.2816, 11.0735)
  line L98 (-115.1907, 10.1247) -> (-115.1907, -6.5098)
  arc A62 (-117.6907, -10.8399) -> (-115.1907, -6.5098) centre (-120.1907, -6.5098) ccw
  line L99 (-117.6907, -10.8399) -> (-121.6189, -13.1079)
  arc A63 (-121.6189, -13.1079) -> (-122.1189, -13.9739) centre (-121.1189, -13.9739) ccw
  line L100 (-122.1189, -13.9739) -> (-122.1189, -15.2165)
  arc A64 (-122.298, -15.4154) -> (-122.1189, -15.2165) centre (-122.3189, -15.2165) ccw
  line L101 (-122.298, -15.4154) -> (-125.1189, -15.7119)
  line L102 (-125.1189, -15.7119) -> (-125.1189, -15.634)
  arc A65 (-125.1189, -15.634) -> (-125.3398, -15.4351) centre (-125.3189, -15.634) ccw
  line L103 (-125.3398, -15.4351) -> (-140.4532, -17.0236)
  arc A66 (-140.4532, -17.0236) -> (-140.6323, -17.2225) centre (-140.4323, -17.2225) ccw
  line L104 (-140.6323, -17.2225) -> (-140.6323, -17.1623)
  arc A67 (-140.8114, -17.3612) -> (-140.6323, -17.1623) centre (-140.8323, -17.1623) ccw
  line L105 (-140.8114, -17.3612) -> (-143.4114, -17.6345)
  spline S2 degree 5 poles (-131.6523, 17.4499) (-131.871, 16.8829) (-132.3693, 15.5934) (-133.1481, 13.5859) (-134.2095, 10.8681) (-135.5564, 7.4521) (-136.9701, 3.9054) (-138.3903, 0.385) (-139.8173, -3.108) (-141.2507, -6.5745) (-142.5604, -9.7063) (-143.5856, -12.1354) (-144.3238, -13.8732) (-144.7729, -14.9268) (-144.9323, -15.3) knots -0.978339 -0.978339 -0.978339 -0.978339 -0.978339 -0.978339 -0.9 -0.8 -0.7 -0.6 -0.5 -0.4 -0.3 -0.2 -0.1 -0.045074 -0.045074 -0.045074 -0.045074 -0.045074 -0.045074
  line L106 (-144.9323, -15.3) -> (-147.3323, -15.3)
  spline S3 degree 3 poles (-147.3323, -15.3) (-147.3606, -15.2315) (-147.3889, -15.163) (-147.4174, -15.0945) (-147.7999, -14.1733) (-148.2003, -13.2596) (-148.603, -12.3469) (-149.0343, -11.3694) (-149.4682, -10.3932) (-149.9035, -9.4176) (-150.1094, -8.9559) (-150.3157, -8.4943) (-150.5222, -8.0328) knots 80.396364 80.396364 80.396364 80.396364 80.841267 80.841267 80.841267 86.826165 86.826165 86.826165 93.23622 93.23622 93.23622 96.269727 96.269727 96.269727 96.269727
  spline S4 degree 5 poles (-150.5222, -8.0328) (-150.5836, -7.8891) (-150.9212, -7.0983) (-151.5369, -5.6459) (-152.4351, -3.5002) (-153.6231, -0.6091) (-155.0461, 2.9325) (-156.4844, 6.5848) (-157.7568, 9.8732) (-158.7459, 12.4635) (-159.4459, 14.3123) (-159.8529, 15.3927) (-159.9652, 15.6911) knots -0.722257 -0.722257 -0.722257 -0.722257 -0.722257 -0.722257 -0.7 -0.6 -0.5 -0.4 -0.3 -0.2 -0.1 -0.061951 -0.061951 -0.061951 -0.061951 -0.061951 -0.061951
  line L107 (-159.9652, 15.6911) -> (-160.6285, 17.4538)
  arc A68 (-160.1605, 18.1298) -> (-160.6285, 17.4538) centre (-160.1605, 17.6298) ccw
  line L108 (-160.1605, 18.1298) -> (-132.1188, 18.1298)
  arc A69 (-131.6523, 17.4499) -> (-132.1188, 18.1298) centre (-132.1188, 17.6298) ccw
  line L109 (-167.1456, -16.5119) -> (-151.6323, -18.1424)
  line L110 (-151.6323, -18.1424) -> (-151.6323, -18.0645)
  arc A70 (-151.4114, -17.8656) -> (-151.6323, -18.0645) centre (-151.4323, -18.0645) ccw
  line L111 (-151.4114, -17.8656) -> (-148.8114, -18.1389)
  arc A71 (-148.6323, -18.3378) -> (-148.8114, -18.1389) centre (-148.8323, -18.3378) ccw
  line L112 (-148.6323, -18.3378) -> (-148.6323, -19.4356)
  arc A72 (-148.8532, -19.6345) -> (-148.6323, -19.4356) centre (-148.8323, -19.4356) ccw
  line L113 (-148.8532, -19.6345) -> (-151.4532, -19.3612)
  arc A73 (-151.6323, -19.1623) -> (-151.4532, -19.3612) centre (-151.4323, -19.1623) ccw
  line L114 (-151.6323, -19.1623) -> (-151.6323, -19.0424)
  line L115 (-151.6323, -19.0424) -> (-167.1456, -17.4119)
  line L116 (-167.1456, -17.4119) -> (-167.1456, -17.4898)
  arc A74 (-167.3665, -17.6887) -> (-167.1456, -17.4898) centre (-167.3456, -17.4898) ccw
  line L117 (-167.3665, -17.6887) -> (-169.9665, -17.4154)
  arc A75 (-170.1456, -17.2165) -> (-169.9665, -17.4154) centre (-169.9456, -17.2165) ccw
  line L118 (-170.1456, -17.2165) -> (-170.1456, -16.1187)
  arc A76 (-169.9247, -15.9198) -> (-170.1456, -16.1187) centre (-169.9456, -16.1187) ccw
  line L119 (-169.9247, -15.9198) -> (-167.3247, -16.1931)
  arc A77 (-167.1456, -16.392) -> (-167.3247, -16.1931) centre (-167.3456, -16.392) ccw
  line L120 (-167.1456, -16.392) -> (-167.1456, -16.5119)
  arc A78 (-123.4224, 7.043) -> (-122.93, 6.6298) centre (-122.93, 7.1298) ccw
  line L121 (-123.4224, 7.043) -> (-126.0097, 21.7167)
  arc A79 (-126.0097, 21.7167) -> (-126.5021, 22.1298) centre (-126.5021, 21.6298) ccw
  line L122 (-126.5021, 22.1298) -> (-165.663, 22.1298)
  arc A80 (-165.663, 22.1298) -> (-166.1554, 21.7167) centre (-165.663, 21.6298) ccw
  line L123 (-166.1554, 21.7167) -> (-168.7428, 7.043)
  arc A81 (-169.2352, 6.6298) -> (-168.7428, 7.043) centre (-169.2352, 7.1298) ccw
  line L124 (-169.2352, 6.6298) -> (-176.588, 6.6298)
  arc A82 (-177.088, 7.1298) -> (-176.588, 6.6298) centre (-176.588, 7.1298) ccw
  line L125 (-177.088, 7.1298) -> (-177.088, 23.1298)
  arc A83 (-176.588, 23.6298) -> (-177.088, 23.1298) centre (-176.588, 23.1298) ccw
  line L126 (-176.588, 23.6298) -> (-121.7059, 23.6298)
  arc A84 (-121.2059, 23.1298) -> (-121.7059, 23.6298) centre (-121.7059, 23.1298) ccw
  line L127 (-121.2059, 23.1298) -> (-121.2059, 7.1298)
  arc A85 (-121.7059, 6.6298) -> (-121.2059, 7.1298) centre (-121.7059, 7.1298) ccw
  line L128 (-121.7059, 6.6298) -> (-122.93, 6.6298)
  arc A86 (-143.6323, -19.4356) -> (-143.4114, -19.6345) centre (-143.4323, -19.4356) ccw
  line L129 (-143.6323, -19.4356) -> (-143.6323, -18.3378)
  arc A87 (-143.4532, -18.1389) -> (-143.6323, -18.3378) centre (-143.4323, -18.3378) ccw
  line L130 (-143.4532, -18.1389) -> (-140.6323, -17.8424)
  line L131 (-140.6323, -17.8424) -> (-140.6323, -17.9203)
  arc A88 (-140.6323, -17.9203) -> (-140.4114, -18.1192) centre (-140.4323, -17.9203) ccw
  line L132 (-140.4114, -18.1192) -> (-125.298, -16.5307)
  arc A89 (-125.298, -16.5307) -> (-125.1189, -16.3318) centre (-125.3189, -16.3318) ccw
  line L133 (-125.1189, -16.3318) -> (-125.1189, -16.2119)
  line L134 (-125.1189, -16.2119) -> (-122.3398, -15.9198)
  arc A90 (-122.1189, -16.1187) -> (-122.3398, -15.9198) centre (-122.3189, -16.1187) ccw
  line L135 (-122.1189, -16.1187) -> (-122.1189, -17.2165)
  arc A91 (-122.298, -17.4154) -> (-122.1189, -17.2165) centre (-122.3189, -17.2165) ccw
  line L136 (-122.298, -17.4154) -> (-125.1189, -17.7119)
  line L137 (-125.1189, -17.7119) -> (-125.1189, -17.634)
  arc A92 (-125.1189, -17.634) -> (-125.3398, -17.4351) centre (-125.3189, -17.634) ccw
  line L138 (-125.3398, -17.4351) -> (-140.4532, -19.0236)
  arc A93 (-140.4532, -19.0236) -> (-140.6323, -19.2225) centre (-140.4323, -19.2225) ccw
  line L139 (-140.6323, -19.2225) -> (-140.6323, -19.2524)
  arc A94 (-140.7218, -19.3518) -> (-140.6323, -19.2524) centre (-140.7323, -19.2524) ccw
  line L140 (-140.7218, -19.3518) -> (-143.4114, -19.6345)
  arc A95 (-143.6323, -21.4356) -> (-143.4114, -21.6345) centre (-143.4323, -21.4356) ccw
  line L141 (-143.6323, -21.4356) -> (-143.6323, -20.3378)
  arc A96 (-143.4532, -20.1389) -> (-143.6323, -20.3378) centre (-143.4323, -20.3378) ccw
  line L142 (-143.4532, -20.1389) -> (-140.6323, -19.8424)
  line L143 (-140.6323, -19.8424) -> (-140.6323, -19.9203)
  arc A97 (-140.6323, -19.9203) -> (-140.4114, -20.1192) centre (-140.4323, -19.9203) ccw
  line L144 (-140.4114, -20.1192) -> (-125.298, -18.5307)
  arc A98 (-125.298, -18.5307) -> (-125.1189, -18.3318) centre (-125.3189, -18.3318) ccw
  line L145 (-125.1189, -18.3318) -> (-125.1189, -18.2119)
  line L146 (-125.1189, -18.2119) -> (-122.3398, -17.9198)
  arc A99 (-122.1189, -18.1187) -> (-122.3398, -17.9198) centre (-122.3189, -18.1187) ccw
  line L147 (-122.1189, -18.1187) -> (-122.1189, -19.2165)
  arc A100 (-122.298, -19.4154) -> (-122.1189, -19.2165) centre (-122.3189, -19.2165) ccw
  line L148 (-122.298, -19.4154) -> (-125.1189, -19.7119)
  line L149 (-125.1189, -19.7119) -> (-125.1189, -19.634)
  arc A101 (-125.1189, -19.634) -> (-125.3398, -19.4351) centre (-125.3189, -19.634) ccw
  line L150 (-125.3398, -19.4351) -> (-140.4532, -21.0236)
  arc A102 (-140.4532, -21.0236) -> (-140.6323, -21.2225) centre (-140.4323, -21.2225) ccw
  line L151 (-140.6323, -21.2225) -> (-140.6323, -21.2524)
  arc A103 (-140.7218, -21.3518) -> (-140.6323, -21.2524) centre (-140.7323, -21.2524) ccw
  line L152 (-140.7218, -21.3518) -> (-143.4114, -21.6345)
  line L153 (-122.1189, -20.1187) -> (-122.1189, -15.2165)
  line L154 (-120.2059, 23.6298) -> (-121.7059, 23.6298)
  line L155 (-176.588, 23.6298) -> (-178.088, 23.6298)
  line L156 (-170.1456, -20.1187) -> (-170.1456, -15.2165)
  line L157 (-184.9592, 2.6298) -> (-184.9592, 6.6298)
  arc A104 (-115.1907, 10.1247) -> (-115.2816, 11.0735) centre (-120.1907, 10.1247) ccw
  constraint coincident A17.start L32.start
  constraint coincident L100.end A64.end
  constraint coincident A60.start L96.start
  constraint coincident L126.end A84.end
  constraint coincident A83.start L126.start
  constraint coincident L42.end A27.end
  constraint coincident L15.end A2.end
  constraint coincident A41.start L73.start
  constraint coincident A33.start L63.start
  constraint coincident L44 L157.end
  constraint perpendicular L44 L157
extrude "Extrude5" add sketch "Sketch6" along normal blind 2 contours L0 L1 L2 L3 L4 L5 L6 L7 L8 L9 L10 L11 A0 L12 L13 L14 A1 L15 L73 A42 L74 A43 L75 L76 L86 L118 L156 | L44 A29 L45 A30 L46 L47 A31 L48 A32 L49 L50 L51 L52 L53 L54 L55 L56 L57 L58 L59 L60 L61 L62 A33 L157 | L32 A18 L33 L34 L35 A19 A20 L36 A21 L37 A22 A23 L38 A24 L39 L40 A25 L41 A26 L42 L96 A61 L97 L98 A62 L99 A63 L100 L126 L135 L147 L153 L154 L155 A104
sketch "Sketch7" plane through (0, 0, 7) normal (0, 0, 1) x (-1, 0, 0)
  line L0 (-178.6113, 1.6298) -> (-178.6113, 23.6298)
  line L1 (-178.6113, 23.6298) -> (-118.121, 23.6298)
  arc A0 (-117.6301, 23.2247) -> (-118.121, 23.6298) centre (-118.121, 23.1298) ccw
  line L2 (-117.6301, 23.2247) -> (-115.2816, 11.0735)
  arc A1 (-115.1907, 10.1247) -> (-115.2816, 11.0735) centre (-120.1907, 10.1247) ccw
  line L3 (-115.1907, 10.1247) -> (-115.1907, -6.5098)
  arc A2 (-117.6907, -10.8399) -> (-115.1907, -6.5098) centre (-120.1907, -6.5098) ccw
  line L4 (-117.6907, -10.8399) -> (-121.6189, -13.1079)
  arc A3 (-121.6189, -13.1079) -> (-122.1189, -13.9739) centre (-121.1189, -13.9739) ccw
  line L5 (-122.1189, -13.9739) -> (-122.1189, -23.408)
  arc A4 (-122.6074, -23.9078) -> (-122.1189, -23.408) centre (-122.6189, -23.408) ccw
  line L6 (-122.6074, -23.9078) -> (-142.1438, -24.3589)
  line L7 (-142.1438, -24.3589) -> (-142.6323, -24.3589)
  line L8 (-142.6323, -24.3589) -> (-142.6323, -24.3702)
  line L9 (-142.6323, -24.3702) -> (-149.6323, -24.3702)
  line L10 (-149.6323, -24.3702) -> (-169.6572, -23.9078)
  arc A5 (-170.1456, -23.408) -> (-169.6572, -23.9078) centre (-169.6456, -23.408) ccw
  line L11 (-170.1456, -23.408) -> (-170.1456, -13.9739)
  arc A6 (-170.1456, -13.9739) -> (-170.6456, -13.1079) centre (-171.1456, -13.9739) ccw
  line L12 (-170.6456, -13.1079) -> (-173.5, -11.4599)
  arc A7 (-176, -7.1298) -> (-173.5, -11.4599) centre (-171, -7.1298) ccw
  line L13 (-176, -7.1298) -> (-176, 1.6298)
  line L14 (-176, 1.6298) -> (-178.6113, 1.6298)
  circle A8 centre (-11.002, 0.0641) radius 7.5
  line L15 (-182.6113, -5.2083) -> (-183.6113, -6.9403)
  line L16 (-183.6113, -6.9403) -> (-182.6113, -8.6724)
  line L17 (-182.6113, -8.6724) -> (-183.6113, -10.4044)
  line L18 (-183.6113, -10.4044) -> (-182.6113, -12.1365)
  line L19 (-182.6113, -12.1365) -> (-183.6113, -13.8685)
  line L20 (-183.6113, -13.8685) -> (-182.6113, -15.6006)
  line L21 (-182.6113, -15.6006) -> (-183.6113, -17.3326)
  line L22 (-183.6113, -17.3326) -> (-182.6113, -19.0647)
  line L23 (-182.6113, -19.0647) -> (-183.6113, -20.7967)
  line L24 (-183.6113, -20.7967) -> (-179.9574, -28.2505)
  arc A9 (-179.9574, -28.2505) -> (-178.1615, -29.3702) centre (-178.1615, -27.3702) ccw
  line L25 (-178.1615, -29.3702) -> (-117.7597, -29.3702)
  arc A10 (-117.7597, -29.3702) -> (-113.1229, -26.2409) centre (-117.7597, -24.3702) ccw
  arc A11 (-89.3732, -10.2649) -> (-113.1229, -26.2409) centre (-89.45, -35.7917) ccw
  line L26 (-89.3732, -10.2649) -> (-11.704, -12.452)
  arc A12 (-11.704, -12.452) -> (-11.9433, 12.5645) centre (-11.002, 0.0641) ccw
  line L27 (-11.9433, 12.5645) -> (-80.6073, 9.9709)
  arc A13 (-112.7407, 25.7315) -> (-80.6073, 9.9709) centre (-80.1774, 51.4853) ccw
  arc A14 (-112.7407, 25.7315) -> (-116.6624, 27.6298) centre (-116.6624, 22.6298) ccw
  line L28 (-116.6624, 27.6298) -> (-197.169, 27.6298)
  arc A15 (-197.169, 27.6298) -> (-202.169, 22.6429) centre (-197.169, 22.6298) ccw
  line L29 (-202.169, 22.6429) -> (-202.2039, 9.25)
  line L30 (-202.2039, 9.25) -> (-186.5961, 9.1821)
  arc A16 (-186.5961, 9.1821) -> (-186.1089, 9.5607) centre (-186.5939, 9.6821) ccw
  line L31 (-186.1089, 9.5607) -> (-183.6113, 19.5409)
  line L32 (-183.6113, 19.5409) -> (-183.6113, -0.0121)
  line L33 (-183.6113, -0.0121) -> (-182.6113, -1.7442)
  line L34 (-182.6113, -1.7442) -> (-183.6113, -3.4762)
  line L35 (-183.6113, -3.4762) -> (-182.6113, -5.2083)
  line L36 (-21.1868, -7.183) -> (-81.002, -5.4987)
  line L37 (-81.002, 4.9525) -> (-21.2587, 7.2091)
  line L38 (-81.002, 4.9525) -> (-81.002, -5.4987)
  arc A17 (-21.2587, 7.2091) -> (-21.1868, -7.183) centre (-11.002, 0.0641) ccw
  dimension "d169" = 25
  dimension "d170" = 5
  dimension "d171" = 5
  dimension "d174" = 70
  constraint concentric A8 A17
  constraint parallel L26 L36
  constraint parallel L27 L37
  constraint vertical L38
  measures "d169" diameter of A17
  measures "d170" distance of L26 L36
  measures "d171" distance of L27 L37
  measures "d174" distance of A8.centre L38
extrude "Extrude6" cut sketch "Sketch7" against normal blind 1 contours L36 L37 L38 A17